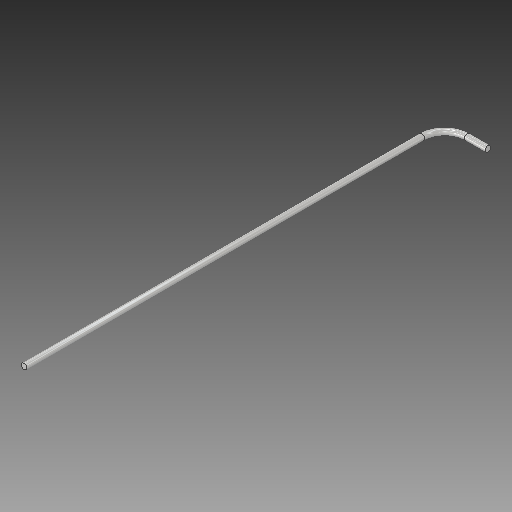
# Autodesk Inventor part: rightFront_tube
Saved by Autodesk Inventor 2019 (Build 230136000, 136)
## iProperties
Created: 2018-07-10
Part Number: rightFront_tube
Material: Generic
Document SubType Name: Modeling
Designer: User
Density: 1 g/cm^3
Appearance: Aluminum - Polished
Author: User
Autodesk Inventor part; units mm, degrees
ref_plane "XZ Plane" through (0, 0, 0) normal (0, 1, 0) x (-1, 0, 0)
ref_plane "XY Plane" through (0, 0, 0) normal (0, 0, 1) x (1, 0, 0)
sketch "Sketch2" plane through (0, 0, 0) normal (0, 0, 1) x (1, 0, 0)
  circle A0 centre (0, 0) radius 9.525
  dimension "d3" = 19.05
  constraints: 1 centre point, 1 coincident
  measures "d3" diameter of A0
extrude "Extrusion2" add sketch "Sketch2" against normal blind 1339.85
ref_plane "Work Plane1" through (76.2, 0, 0) normal (1, 0, 0) x (0, 1, 0)
sketch "Sketch9" plane through (76.2, 0, 0) normal (1, 0, 0) x (0, 1, 0)
  line L0 (-9.525, -1339.85) -> (9.525, -1339.85) projected
  circle A0 centre (0, -1416.05) radius 9.525
  line L1 (0, -1339.85) -> (0, -1416.05) construction
  point P0 (0, 0)
  dimension "d17" = 19.05
  dimension "d18" = 76.2
  constraints: 2 end point, 1 centre point, 1 midpoint, 1 perpendicular
  measures "d17" diameter of A0
  measures "d18" distance of L1.start L1.end
extrude "Extrusion4" add sketch "Sketch9" along normal blind 69.85
sketch "Sketch11" plane through (0, 0, -1339.85) normal (0, 0, -1) x (-1, 0, 0)
  circle A0 centre (0, 0) radius 9.525 projected
sketch "Sketch12" plane through (0, 0, 0) normal (0, 1, 0) x (-1, 0, 0)
  line L0 (-76.2, -1425.575) -> (-76.2, -1406.525) projected
  line L1 (-9.525, -1339.85) -> (9.525, -1339.85) projected
  arc A0 (-76.2, -1416.05) -> (0, -1339.85) centre (-76.2, -1339.85) ccw
  point P0 (0, 0)
  dimension "d21" = 76.2
  constraints: 2 midpoint, 2 point on circle, 1 centre point
  measures "d21" radius of A0
sweep "Sweep2" add profiles "Sketch11" path "Sketch12" path curves A0
equation "\"d3\" = tubeD"
equation "\"d17\" = tubeD"
equation "\"d18\" = tubeTurnR"
equation "\"d21\" = tubeTurnR"
equation "\"d4\" = tubeTurnR"
equation "\"wallThick\" = 44.45"
equation "\"roomWidth\" = 3048"
equation "\"roomDepth\" = 3657.6"
equation "\"roomHeight\" = 2438.4"
equation "\"doorWidth\" = 895.35"
equation "\"doorHeight\" = 2108.2"
equation "\"doorX\" = 774.7"
equation "\"doorY\" = 88.9"
equation "\"doorLip\" = 76.2"
equation "\"doorThick\" = 57.15"
equation "\"tubeTurnR\" = 76.2"
equation "\"tubeD\" = 19.05"
body "Solid2"
